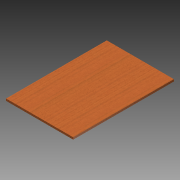
# Autodesk Inventor part: top plate
Saved by Autodesk Inventor 2015 SP1 (Build 190203100, 203)
## iProperties
Created: 2015-04-22
Part Number: top plate
Material: Wood (Cherry)
Document SubType Name: Modeling
Designer: ubik
Density: 0.63 g/cm^3
Appearance: Cherry - Natural Low Gloss
Author: ubik
Autodesk Inventor part; units mm, degrees
ref_plane "YZ Plane" through (0, 0, 0) normal (1, 0, 0) x (0, 1, 0)
ref_plane "XZ Plane" through (0, 0, 0) normal (0, 1, 0) x (-1, 0, 0)
ref_plane "XY Plane" through (0, 0, 0) normal (0, 0, 1) x (1, 0, 0)
sketch "Sketch1" plane through (0, 0, 0) normal (0, 0, 1) x (1, 0, 0)
  line L0 (0, 0) -> (400, 0)
  line L1 (400, 0) -> (400, 600)
  line L2 (400, 600) -> (0, 600)
  line L3 (0, 600) -> (0, 0)
  dimension "d0" = 400
  dimension "d1" = 600
  constraints: 8 end point, 2 parallel, 1 horizontal, 1 perpendicular
  measures "d0" distance of L2.end L1.end
  measures "d1" distance of L1.end L0.end
extrude "Extrusion1" add sketch "Sketch1" along normal blind 12
hole "Hole1" [suppressed]
pattern_linear "Rectangular Pattern1" [suppressed]
sketch "Sketch2" plane through (0, 0, 12) normal (0, 0, 1) x (1, 0, 0)
  line L0 (400, 60) -> (370, 60)
  line L1 (370, 60) -> (370, 30)
  line L2 (370, 30) -> (400, 30)
  line L3 (400, 30) -> (400, 60)
  line L4 (0, 0) -> (400, 0) projected
  line L5 (400, 0) -> (400, 600) projected
  dimension "d28" = 30
  dimension "d29" = 30
  dimension "d30" = 30
  dimension "d33" = 0
  constraints: 8 end point, 2 parallel, 1 horizontal, 1 perpendicular
  measures "d28" distance of L2.end L1.end
  measures "d29" distance of L0.end L1.end
  measures "d30" distance between parallel lines of L4 L2
  measures "d33" distance between parallel lines of L5 L3
extrude "Extrusion2" [suppressed]
body "Solid1"
